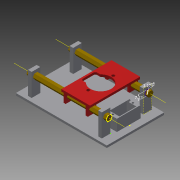
# Autodesk Inventor part: rotate-bot-base
Saved by Autodesk Inventor 2015 SP2 (Build 190223200, 223)
## iProperties
Created: 2015-05-24
Part Number: rotate-bot-base
Material: Generic
Document SubType Name: Modeling
Designer: caleb
Density: 1 g/cm^3
Appearance: Default
Author: caleb
Autodesk Inventor part; units mm, degrees
sketch "Sketch1" plane through (0, 0, 0) normal (0, 0, 1) x (1, 0, 0)
  line L0 (-63.5, -40) -> (63.5, -40)
  line L1 (63.5, -40) -> (63.5, 40)
  line L2 (63.5, 40) -> (-63.5, 40)
  line L3 (-63.5, 40) -> (-63.5, -40)
  line L4 (-63.5, -40) -> (63.5, 40) construction
  line L5 (63.5, -40) -> (-63.5, 40) construction
  point P0 (0, 0)
  dimension "d0" = 80
  dimension "d19" = 127
  constraints: 12 end point, 2 midpoint, 2 parallel, 1 horizontal, 1 perpendicular
  measures "d0" distance of L0.end L1.end
  measures "d19" distance of L1.end L2.end
extrude "Extrusion1" add sketch "Sketch1" against normal blind 3
sketch "Sketch2" plane through (0, 0, 0) normal (0, 0, 1) x (1, 0, 0)
  line L0 (-63.5, -40) -> (63.5, -40) projected
  line L1 (63.5, -40) -> (63.5, 40) projected
  line L2 (63.5, 40) -> (-63.5, 40) projected
  line L3 (-63.5, 40) -> (-63.5, -40) projected
  line L4 (46.5, 23) -> (51.5, 23)
  line L5 (51.5, 23) -> (51.5, 35)
  line L6 (51.5, 35) -> (46.5, 35)
  line L7 (46.5, 35) -> (46.5, 23)
  line L8 (46.5, 23) -> (51.5, 35) construction
  line L9 (51.5, 23) -> (46.5, 35) construction
  line L10 (-51.5, 23) -> (-46.5, 23)
  line L11 (-46.5, 23) -> (-46.5, 35)
  line L12 (-46.5, 35) -> (-51.5, 35)
  line L13 (-51.5, 35) -> (-51.5, 23)
  line L14 (-51.5, 23) -> (-46.5, 35) construction
  line L15 (-46.5, 23) -> (-51.5, 35) construction
  line L16 (-49, 29) -> (49, 29) construction
  point P0 (0, 0)
  point P1 (49, 29)
  point P2 (0, 29)
  dimension "d3" = 12
  dimension "d5" = 5
  dimension "d48" = 12
  dimension "d49" = 5
  constraints: 26 end point, 7 midpoint, 4 parallel, 3 perpendicular, 2 equal length, 2 horizontal, 1 horizontal alignment, 1 vertical alignment
  measures "d3" distance of L4.end L5.end
  measures "d5" distance of L4.start L4.end
  measures "d48" distance between parallel lines of L1 L5
  measures "d49" distance between parallel lines of L2 L6
extrude "Extrusion2" add sketch "Sketch2" along normal blind 31.5 contours L7 L6 L5 L4 | L13 L12 L11 L10
sketch "Sketch3" plane through (51.5, 23, 0) normal (1, 0, 0) x (0, 0, -1)
  circle A0 centre (-23.885, 6) radius 1.5875 construction
  line L0 (0, 12) -> (0, 0) construction
  line L1 (0, 12) -> (-31.5, 12) construction
  line L2 (-31.5, 0) -> (-31.5, 12) construction
  line L3 (0, 0) -> (-31.5, 0) construction
  line L4 (-27.5, 8.0871) -> (-23.885, 10.1742)
  line L5 (-23.885, 10.1742) -> (-20.27, 8.0871)
  line L6 (-20.27, 8.0871) -> (-20.27, 3.9129)
  line L7 (-20.27, 3.9129) -> (-23.885, 1.8258)
  line L8 (-23.885, 1.8258) -> (-27.5, 3.9129)
  line L9 (-27.5, 3.9129) -> (-27.5, 8.0871)
  point P0 (0, -46)
  point P1 (-31.5, 6)
  dimension "d9" = 3.175
  dimension "pencil_d" = 7.23
  dimension "d51" = 4
  constraints: 12 end point, 1 centre point, 1 coincident, 1 horizontal alignment, 1 midpoint, 1 vertical, 13 other
  measures "d9" diameter of A0
  measures "pencil_d" distance between parallel lines of L6 L9
  measures "d51" distance from line of point (-31.5, 6) L9
extrude "Extrusion3" cut sketch "Sketch3" against normal through all
extrude "Extrusion4" add sketch "Sketch3" along normal blind 4 separate body
ref_plane "Work Plane1" through (-55.5, 23, 0) normal (-1, 0, 0) x (0, 0, 1)
extrude "Extrusion5" add sketch "Sketch3" against normal up to surface (107 mm away) bodies 2
mirror "Mirror1" about plane through (0, 0, 0) normal (0, 1, 0) of "Extrusion2", "Extrusion3" bodies 1
mirror "Mirror2" about plane through (0, 0, 0) normal (0, 1, 0) bodies 2
ref_plane "Work Plane2" through (0, 0, 31.5) normal (0, 0, 1) x (1, 0, 0)
sketch "Sketch4" plane through (0, 0, 31.5) normal (0, 0, 1) x (1, 0, 0)
  line L0 (-51.5, 23) -> (-46.5, 23) construction
  line L1 (-46.5, 23) -> (-46.5, 35) construction
  line L2 (-46.5, 35) -> (-51.5, 35) construction
  line L3 (-51.5, 35) -> (-51.5, 23) construction
  line L4 (46.5, 23) -> (51.5, 23) construction
  line L5 (51.5, 23) -> (51.5, 35) construction
  line L6 (51.5, 35) -> (46.5, 35) construction
  line L7 (46.5, 35) -> (46.5, 23) construction
  line L8 (46.5, -23) -> (51.5, -23) construction
  line L9 (46.5, -35) -> (46.5, -23) construction
  line L10 (51.5, -35) -> (46.5, -35) construction
  line L11 (51.5, -23) -> (51.5, -35) construction
  line L12 (-51.5, -23) -> (-46.5, -23) construction
  line L13 (-51.5, -35) -> (-51.5, -23) construction
  line L14 (-46.5, -35) -> (-51.5, -35) construction
  line L15 (-46.5, -23) -> (-46.5, -35) construction
  line L16 (-5, -35) -> (35, -35)
  line L17 (35, -35) -> (35, 35)
  line L18 (35, 35) -> (-5, 35)
  line L19 (-5, 35) -> (-5, -35)
  line L20 (-5, -35) -> (35, 35) construction
  line L21 (35, -35) -> (-5, 35) construction
  point P0 (0, 0)
  point P1 (15, 0)
  point P2 (15, 0)
  dimension "d23" = 40
  dimension "d24" = 15
  constraints: 12 end point, 3 midpoint, 2 parallel, 1 collinear, 1 horizontal, 1 horizontal alignment, 1 perpendicular
  measures "d23" distance of L16.start L16.end
  measures "d24" distance of point (0, 0) point (15, 0)
extrude "Extrusion6" add sketch "Sketch4" against normal blind 3 separate body
sketch "Sketch5" plane through (0, 0, 28.5) normal (0, 0, -1) x (-1, 0, 0)
  line L0 (5, -35) -> (-35, -35) construction
  line L1 (-35, -35) -> (-35, 35) construction
  line L2 (-35, 35) -> (5, 35) construction
  line L3 (5, 35) -> (5, -35) construction
  line L4 (-32, 23) -> (-29, 23)
  line L5 (-29, 23) -> (-29, 35)
  line L6 (-29, 35) -> (-32, 35)
  line L7 (-32, 35) -> (-32, 23)
  line L8 (-32, 23) -> (-29, 35) construction
  line L9 (-29, 23) -> (-32, 35) construction
  line L10 (-46.5, 35) -> (-51.5, 35) projected
  line L11 (-51.5, 35) -> (-46.5, 35) projected
  line L12 (-46.5, 24.8258) -> (-46.5, 26.9129) projected
  point P0 (0, 0)
  point P1 (-51.5, 29)
  point P2 (-30.5, 29)
  point P3 (-30.5, 29)
  dimension "d27" = 3
  dimension "d29" = 3
  constraints: 12 end point, 3 midpoint, 2 parallel, 1 collinear, 1 horizontal, 1 horizontal alignment, 1 perpendicular
  measures "d27" distance between parallel lines of L1 L7
  measures "d29" distance of L4.start L4.end
extrude "Extrusion7" add sketch "Sketch5" along normal blind 12 bodies 3
extrude "Extrusion8" cut sketch "Sketch3" against normal through all bodies 3
ref_plane "Work Plane3" through (15, -35, 31.5) normal (1, 0, 0) x (0, 0, -1)
ref_plane "Work Plane4" through (-5, 0, 31.5) normal (0, 1, 0) x (1, 0, 0)
mirror "Mirror3" about plane through (15, -35, 31.5) normal (1, 0, 0) of "Extrusion7", "Extrusion8" bodies 3
mirror "Mirror4" about plane through (-5, 0, 31.5) normal (0, 1, 0) of "Extrusion7", "Extrusion8", "Mirror3" bodies 3
sketch "Sketch7" plane through (0, 0, 31.5) normal (0, 0, 1) x (1, 0, 0)
  circle A0 centre (15, -17.5) radius 2 projected
  circle A1 centre (15, 17.5) radius 2 projected
  arc A2 (11.45, 13.5424) -> (11.45, -13.5424) centre (15, 0) ccw projected
  line L0 (11.45, -17.5) -> (11.45, -13.5424) projected
  arc A3 (11.45, -17.5) -> (18.55, -17.5) centre (15, -17.5) ccw projected
  line L1 (18.55, -13.5424) -> (18.55, -17.5) projected
  arc A4 (18.55, -13.5424) -> (18.55, 13.5424) centre (15, 0) ccw projected
  line L2 (18.55, 13.5424) -> (18.55, 17.5) projected
  arc A5 (18.55, 17.5) -> (11.45, 17.5) centre (15, 17.5) ccw projected
  line L3 (11.45, 17.5) -> (11.45, 13.5424) projected
  circle A6 centre (22.55, 0) radius 4.55 projected
  arc A7 (10.95, 13.9229) -> (10.95, -13.9229) centre (15, 0) ccw
  line L4 (10.95, 13.9229) -> (10.95, 17.5)
  arc A8 (19.05, 17.5) -> (10.95, 17.5) centre (15, 17.5) ccw
  line L5 (19.05, 17.5) -> (19.05, 13.9229)
  arc A9 (19.05, -13.9229) -> (19.05, 13.9229) centre (15, 0) ccw
  line L6 (19.05, -13.9229) -> (19.05, -17.5)
  arc A10 (10.95, -17.5) -> (19.05, -17.5) centre (15, -17.5) ccw
  line L7 (10.95, -17.5) -> (10.95, -13.9229)
  point P0 (0, 0)
  dimension "d39" = 0.5
  constraints: 8 end point, 8 point on circle, 4 centre point, 7 other
  measures "d39" distance between parallel lines of L3 L4
extrude "Extrusion10" cut sketch "Sketch7" against normal blind 0.001 contours L3 A5 L2 A4 L1 A3 L0 A2 | L4 A8 L5 A9 L6 A10 L7 A7 bodies 3
sketch "Sketch8" plane through (0, 0, 31.499) normal (0, 0, 1) x (1, 0, 0)
  circle A0 centre (22.55, 0) radius 4.55 construction
  circle A1 centre (15, 17.5) radius 2 construction
  circle A2 centre (15, -17.5) radius 2 construction
  arc A3 (10.95, 13.9229) -> (10.95, -13.9229) centre (15, 0) ccw construction
  line L0 (10.95, -17.5) -> (10.95, -13.9229) construction
  arc A4 (10.95, -17.5) -> (19.05, -17.5) centre (15, -17.5) ccw construction
  line L1 (19.05, -13.9229) -> (19.05, -17.5) construction
  arc A5 (19.05, -13.9229) -> (19.05, 13.9229) centre (15, 0) ccw construction
  line L2 (19.05, 17.5) -> (19.05, 13.9229) construction
  arc A6 (19.05, 17.5) -> (10.95, 17.5) centre (15, 17.5) ccw construction
  line L3 (10.95, 13.9229) -> (10.95, 17.5) construction
  circle A7 centre (15, 0) radius 14.5
  arc A8 (10.95, 13.9229) -> (10.95, -13.9229) centre (15, 0) ccw projected
  point P0 (0, 0)
  constraints: 1 centre point, 1 coincident, 1 concentric
extrude "Extrusion11" cut sketch "Sketch8" along normal through all both and the other way through all bodies 3
sketch "Sketch9" plane through (15, 17.5, 31.5) normal (0, 0, 1) x (1, 0, 0)
  circle A0 centre (0, 0) radius 2 projected
  circle A1 centre (0, -35) radius 2 projected
  point P0 (-15, -17.5)
extrude "Extrusion12" cut sketch "Sketch9" against normal through all bodies 3
sketch "Sketch11" plane through (0, 0, 31.5) normal (0, 0, 1) x (1, 0, 0)
  arc A0 (3.1784, -7.5) -> (3.1784, 7.5) centre (15, 0) ccw construction
  line L0 (3.1784, -7.5) -> (-2, -7.5) construction
  line L1 (-2, -7.5) -> (-2, 7.5) construction
  line L2 (-2, 7.5) -> (3.1784, 7.5) construction
  arc A1 (2.9066, -8) -> (2.9066, 8) centre (15, 0) ccw construction
  line L3 (2.9066, -8) -> (-2.5, -8)
  line L4 (-2.5, -8) -> (-2.5, 8)
  line L5 (-2.5, 8) -> (2.9066, 8)
  line L6 (46.5, -35) -> (46.5, -23) projected
  line L7 (46.5, -23) -> (51.5, -23) projected
  line L8 (51.5, -23) -> (51.5, -35) projected
  line L9 (51.5, -35) -> (46.5, -35) projected
  line L10 (-51.5, -35) -> (-51.5, -23) projected
  line L11 (-51.5, -23) -> (-46.5, -23) projected
  line L12 (-46.5, -23) -> (-46.5, -35) projected
  line L13 (-46.5, -35) -> (-51.5, -35) projected
  line L14 (46.5, 23) -> (46.5, 35) projected
  line L15 (46.5, 35) -> (51.5, 35) projected
  line L16 (51.5, 35) -> (51.5, 23) projected
  line L17 (51.5, 23) -> (46.5, 23) projected
  line L18 (-51.5, 23) -> (-51.5, 35) projected
  line L19 (-51.5, 35) -> (-46.5, 35) projected
  line L20 (-46.5, 35) -> (-46.5, 23) projected
  line L21 (-46.5, 23) -> (-51.5, 23) projected
  line L22 (-63.5, -40) -> (63.5, -40) projected
  line L23 (63.5, -40) -> (63.5, 40) projected
  line L24 (63.5, 40) -> (-63.5, 40) projected
  line L25 (-63.5, 40) -> (-63.5, -40) projected
  arc A2 (10.95, 13.9229) -> (10.95, -13.9229) centre (15, 0) ccw construction
  line L26 (2.9066, 8) -> (2.9066, -8)
  point P0 (0, 0)
  constraints: 8 end point, 2 point on circle, 1 centre point, 1 concentric, 3 other
extrude "Extrusion13" cut sketch "Sketch11" against normal through all contours L3 L4 L5 L26 bodies 3
sketch "Sketch12" plane through (0, 0, 0) normal (0, 0, 1) x (1, 0, 0)
  circle A0 centre (46.15, 13.8634) radius 1.27 projected
  circle A1 centre (46.15, -14.0766) radius 1.27 projected
  line L0 (52.5, 16.4034) -> (52.5, -16.6166) projected
  line L1 (52.5, -16.6166) -> (39.8, -16.6166) projected
  line L2 (39.8, 16.4034) -> (39.8, -16.6166) projected
  line L3 (52.5, 16.4034) -> (39.8, 16.4034) projected
  line L4 (52.5, -11.5366) -> (39.8, -11.5366) projected
  line L5 (39.8, 11.3234) -> (52.5, 11.3234) projected
  point P0 (0, 0)
extrude "Extrusion14" add sketch "Sketch12" along normal blind 16 contours L0 L5 L2 L3 | L0 L1 L2 L4 bodies 1
sketch "Sketch13" plane through (52.5, -16.6166, 0) normal (1, 0, 0) x (0, 0, -1)
  line L0 (0, 5.08) -> (0, 0) projected
  line L1 (0, 5.08) -> (-16, 5.08) projected
  line L2 (-16, 0) -> (-16, 5.08) projected
  line L3 (0, 0) -> (-16, 0) projected
  line L4 (0, 33.02) -> (0, 27.94) projected
  line L5 (0, 33.02) -> (-16, 33.02) projected
  line L6 (-16, 27.94) -> (-16, 33.02) projected
  line L7 (0, 27.94) -> (-16, 27.94) projected
  line L8 (-16, 5.08) -> (-16, 27.94)
  line L9 (-16, 1.27) -> (-16, 3.81) projected
  line L10 (0, 27.94) -> (0, 5.08)
  line L11 (0, 56.6166) -> (0, -23.3834) projected
  point P0 (0, 16.6166)
  constraints: 4 end point, 2 collinear
ref_plane "Work Plane5" through (46.15, -16.6166, 0) normal (1, 0, 0) x (0, 0, -1)
extrude "Extrusion15" add sketch "Sketch13" along normal blind 1.7 bodies 1
mirror "Mirror5" about plane through (46.15, -16.6166, 0) normal (1, 0, 0) of "Extrusion15" bodies 1
sketch "Sketch14" plane through (0, 0, 16) normal (0, 0, 1) x (1, 0, 0)
  line L0 (39.8, 11.3234) -> (52.5, 11.3234) construction
  line L1 (52.5, 11.3234) -> (52.5, -11.5366) construction
  line L2 (52.5, -11.5366) -> (39.8, -11.5366) construction
  line L3 (39.8, 11.3234) -> (39.8, -11.5366) construction
  circle A0 centre (46.15, -14.0766) radius 1.27 construction
  circle A1 centre (46.15, 13.8634) radius 1.27 construction
  line L4 (38.1, 16.4034) -> (54.2, 16.4034) construction
  line L5 (38.1, 16.4034) -> (38.1, -16.6166) construction
  line L6 (54.2, -16.6166) -> (38.1, -16.6166) construction
  line L7 (54.2, 16.4034) -> (54.2, -16.6166) construction
  line L8 (53, 11.8234) -> (39.3, 11.8234)
  line L9 (39.3, 11.8234) -> (39.3, -12.0366)
  line L10 (39.3, -12.0366) -> (53, -12.0366)
  line L11 (53, -12.0366) -> (53, 11.8234)
  point P0 (0, 0)
  dimension "d56" = 0.5
  constraints: 8 end point, 3 other
  measures "d56" distance between parallel lines of L0 L8
extrude "Extrusion16" cut sketch "Sketch14" against normal up to surface (16 mm away) bodies 1
sketch "Sketch15" plane through (54.2, 16.4034, 16) normal (0, 1, 0) x (1, 0, 0)
  line L0 (-16.1, 16) -> (0, 16) construction
  line L1 (-16.1, 16) -> (-16.1, 0) construction
  line L2 (-16.1, 0) -> (0, 0) construction
  line L3 (0, 16) -> (0, 0) construction
  line L4 (-5.55, 9) -> (-10.55, 9)
  line L5 (-10.55, 9) -> (-10.55, 13)
  line L6 (-10.55, 13) -> (-5.55, 13)
  line L7 (-5.55, 13) -> (-5.55, 9)
  point P0 (-54.2, 16)
  point P1 (-8.05, 13)
  point P2 (-8.05, 16)
  dimension "d59" = 3
  dimension "d61" = 5
  dimension "d62" = 7
  constraints: 8 end point, 2 midpoint, 2 parallel, 1 horizontal, 1 perpendicular, 1 vertical alignment
  measures "d59" distance between parallel lines of L0 L6
  measures "d61" distance of L5.end L6.end
  measures "d62" distance between parallel lines of L4 L0
extrude "Extrusion17" cut sketch "Sketch15" against normal up to surface (4.58 mm away) bodies 1
sketch "Sketch16" plane through (54.2, 16.4034, 16) normal (0, 1, 0) x (1, 0, 0)
  line L0 (-5.55, 9) -> (-10.55, 9) projected
  line L1 (-10.55, 9) -> (-10.55, 13) projected
  line L2 (-10.55, 13) -> (-5.55, 13) projected
  line L3 (-5.55, 13) -> (-5.55, 9) projected
  line L4 (-16.1, 16) -> (0, 16) projected
  line L5 (-16.1, 16) -> (-16.1, 0) projected
  line L6 (-16.1, 0) -> (0, 0) projected
  line L7 (0, 16) -> (0, 0) projected
  line L8 (-10.55, 9) -> (-5.55, 9) projected
  line L9 (-7.7733, 9) -> (-12.1233, 0)
  line L10 (-14.9, 0) -> (-1.2, 0) projected
  line L11 (-10.55, 9) -> (-14.9, 0)
  point P0 (-54.2, 16)
  dimension "d65" = 2.5
  constraints: 4 end point, 2 point on line, 1 parallel
  measures "d65" distance between parallel lines of L11 L9
extrude "Extrusion18" cut sketch "Sketch16" against normal up to surface (28.44 mm away) contours L9 L6 L11 L0 bodies 1
sketch "Sketch17" plane through (54.2, 16.4034, 16) normal (0, 1, 0) x (1, 0, 0)
  line L0 (-14.9, 0) -> (-10.55, 9) projected
  line L1 (-10.55, 9) -> (-10.55, 13) projected
  line L2 (-10.55, 13) -> (-5.55, 13) projected
  line L3 (-5.55, 13) -> (-5.55, 9) projected
  line L4 (-5.55, 9) -> (-7.7733, 9) projected
  line L5 (-7.7733, 9) -> (-12.1233, 0) projected
  line L6 (-12.1233, 0) -> (0, 0) projected
  line L7 (0, 16) -> (0, 0) projected
  line L8 (-16.1, 16) -> (0, 16) projected
  line L9 (-16.1, 16) -> (-16.1, 0) projected
  line L10 (-16.1, 0) -> (-14.9, 0) projected
  line L11 (-5.55, 9) -> (-9.8532, 4.6968)
  point P0 (-54.2, 16)
  dimension "d68" = 45
  constraints: 2 end point, 1 point on line
  measures "d68" angle of L11 L4
extrude "Extrusion19" cut sketch "Sketch17" against normal up to next contours L11 L5 L4 bodies 1
sketch "Sketch18" plane through (55.5, -31.0871, 20.27) normal (1, 0, 0) x (0, 0, -1)
  line L0 (-3.615, -2.0871) -> (-7.23, 0) projected
  line L1 (0, 0) -> (-3.615, -2.0871) projected
  line L2 (0, 4.1742) -> (0, 0) projected
  line L3 (-3.615, 6.2614) -> (0, 4.1742) projected
  line L4 (-7.23, 4.1742) -> (-3.615, 6.2614) projected
  line L5 (-7.23, 0) -> (-7.23, 4.1742) projected
  point P0 (20.27, 31.0871)
  point P1 (-3.615, 2.0871)
  point P2 (-7.23, 2.0871)
  constraints: 1 horizontal alignment, 1 midpoint, 1 vertical alignment
sketch "Sketch20" plane through (0, 0, 31.5) normal (0, 0, 1) x (1, 0, 0)
  line L0 (2.9066, -8) -> (-2.5, -8) projected
  line L1 (-2.5, -8) -> (-2.5, 8) projected
  line L2 (-2.5, 8) -> (2.9066, 8) projected
  arc A0 (10.95, 13.9229) -> (2.9066, 8) centre (15, 0) ccw projected
  line L3 (10.95, 13.9229) -> (10.95, 17.5) projected
  arc A1 (19.05, 17.5) -> (10.95, 17.5) centre (15, 17.5) ccw projected
  line L4 (19.05, 17.5) -> (19.05, 13.9229) projected
  arc A2 (19.05, -13.9229) -> (19.05, 13.9229) centre (15, 0) ccw projected
  line L5 (19.05, -13.9229) -> (19.05, -17.5) projected
  arc A3 (10.95, -17.5) -> (19.05, -17.5) centre (15, -17.5) ccw projected
  line L6 (10.95, -17.5) -> (10.95, -13.9229) projected
  arc A4 (2.9066, -8) -> (10.95, -13.9229) centre (15, 0) ccw projected
  line L7 (-5, -35) -> (35, -35) projected
  line L8 (35, -35) -> (35, 35) projected
  line L9 (35, 35) -> (-5, 35) projected
  line L10 (-5, 35) -> (-5, -35) projected
  line L11 (2.9066, 8) -> (-2.5, 8) projected
  line L12 (-2.5, -8) -> (2.9066, -8) projected
  line L13 (-2.5, -8) -> (-0.5, -10)
  line L14 (-0.5, -10) -> (4.5, -10)
  point P0 (0, 0)
  dimension "d71" = 45
  dimension "d72" = 10
  constraints: 4 end point, 1 horizontal, 1 point on circle
  measures "d71" angle of L0 L13
  measures "d72" distance from line of point (0, 0) L14
extrude "Extrusion20" cut sketch "Sketch20" against normal through all contours A4 L14 L13 L0 bodies 3
mirror "Mirror6" about plane through (-5, 0, 31.5) normal (0, 1, 0) of "Extrusion20" bodies 3
